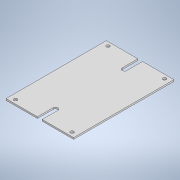
# Autodesk Inventor part: etl standard baseplate with cutouts
Saved by Autodesk Inventor 2022 (Build 260153000, 153)
## iProperties
Created: 2021-07-27
Part Number: etl standard baseplate with cutouts
Material: Generic
Document SubType Name: Modeling
Designer: Caleb
Density: 1 g/cm^3
Appearance: Default
Sending System: Autodesk Inventor 2022
Preprocessor: ST-DEVELOPER v18.1
Title: C:\Users\Caleb\Desktop\etl standard baseplate.stp
Author: Caleb
Autodesk Inventor part; units mm, degrees
ref_plane "YZ Plane" through (0, 0, 0) normal (1, 0, 0) x (0, 1, 0)
ref_plane "XZ Plane" through (0, 0, 0) normal (0, 1, 0) x (-1, 0, 0)
ref_plane "XY Plane" through (0, 0, 0) normal (0, 0, 1) x (1, 0, 0)
sketch "Sketch2" plane through (0, 0, 0) normal (0, 1, 0) x (-1, 0, 0)
  line L0 (-21.55, -32) -> (21.55, -32)
  line L1 (21.55, -32) -> (21.55, 32)
  line L2 (21.55, 32) -> (-21.55, 32)
  line L3 (-21.55, 32) -> (-21.55, -32)
  line L4 (-21.55, -32) -> (21.55, 32) construction
  line L5 (21.55, -32) -> (-21.55, 32) construction
  point P0 (0, 0)
  dimension "d28" = 64
  dimension "d29" = 43.1
  constraints: 12 end point, 2 midpoint, 2 parallel, 1 horizontal, 1 perpendicular
  measures "d28" distance of L0.end L1.end
  measures "d29" distance of L0.start L0.end
extrude "Extrusion2" add sketch "Sketch2" along normal blind 1
sketch "Sketch3" plane through (0, 1, 0) normal (0, 1, 0) x (1, 0, 0)
  point P0 (0, 0)
  point P1 (-18.05, -29.5)
  point P2 (-18.05, 29.5)
  point P3 (18.05, 29.5)
  point P4 (18.05, -29.5)
  dimension "d32" = 59
  dimension "d33" = 29.5
  dimension "d34" = 36.1
  dimension "d35" = 18.05
  constraints: 2 horizontal alignment, 2 vertical alignment
  measures "d32" distance of point (-18.05, 29.5) point (-18.05, -29.5)
  measures "d33" vertical distance of point (-18.05, -29.5) point (0, 0)
  measures "d34" distance of point (-18.05, -29.5) point (18.05, -29.5)
  measures "d35" horizontal distance of point (-18.05, -29.5) point (0, 0)
hole "Hole1" at (-18.05, 1, 29.5) at (-18.05, 1, -29.5) at (18.05, 1, -29.5) at (18.05, 1, 29.5) direction (0, -1, 0) diameter 2.2 end through all clearance for "Flat Head Machine Screw" size "M2" standard "Ansi Metric M Profile"
sketch "Sketch4" plane through (0, 1, 0) normal (0, 1, 0) x (1, 0, 0)
  line L0 (-21.55, -32) -> (21.55, -32) projected
  line L1 (-1.5, -32) -> (-1.5, -22)
  line L2 (1.5, -32) -> (1.5, -22)
  arc A0 (1.5, -22) -> (-1.5, -22) centre (0, -22) ccw
  line L3 (-5.1914, 0) -> (6.1695, 0) construction
  line L4 (-1.5, 32) -> (-1.5, 22)
  line L5 (1.5, 32) -> (1.5, 22)
  arc A1 (-1.5, 22) -> (1.5, 22) centre (0, 22) ccw
  line L6 (21.55, 32) -> (-21.55, 32) projected
  point P0 (0, 0)
  dimension "d43" = 1.5
  dimension "d44" = 3
  dimension "d45" = 10
  dimension "d46" = 1.5
  constraints: 10 end point, 5 symmetric about line, 4 point on circle, 2 centre point, 2 perpendicular, 2 point on line, 1 horizontal, 1 parallel, 1 other
  measures "d43" distance from line of L2 point (0, 0)
  measures "d44" distance between parallel lines of L1 L2
  measures "d45" distance of L1.start L1.end
  measures "d46" radius of A0
extrude "Extrusion3" cut sketch "Sketch4" against normal through all
equation "\"d33\" = 0.5 * d32"
equation "\"d35\" = 0.5 * d34"
body "Solid3"
